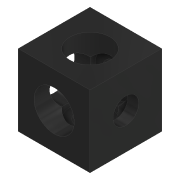
# Autodesk Inventor part: 2020CubeConnector
Saved by Autodesk Inventor 2020 (Build 240168000, 168)
## iProperties
Created: 2021-10-10
Part Number: 2020CubeConnector
Material: Aluminum 6061-AHC
Document SubType Name: Modeling
Designer: Henry Cawley
Density: 2.7 g/cm^3
Appearance: Aluminum - Dark(1)
Author: Henry Cawley
Autodesk Inventor part; units mm, degrees
ref_plane "YZ Plane" through (0, 0, 0) normal (1, 0, 0) x (0, 1, 0)
ref_plane "XZ Plane" through (0, 0, 0) normal (0, 1, 0) x (-1, 0, 0)
ref_plane "XY Plane" through (0, 0, 0) normal (0, 0, 1) x (1, 0, 0)
sketch "Sketch1" plane through (0, 0, 0) normal (1, 0, 0) x (0, 1, 0)
  line L0 (0, 0) -> (20, 0)
  line L1 (20, 0) -> (20, -20)
  line L2 (20, -20) -> (0, -20)
  line L3 (0, -20) -> (0, 0)
  dimension "d0" = 20
  dimension "d1" = 20
  constraints: 8 end point, 2 parallel, 1 horizontal, 1 perpendicular
  measures "d0" distance of L1.end L2.end
  measures "d1" distance of L0.end L1.end
extrude "Extrusion1" add sketch "Sketch1" along normal blind 20
sketch "Sketch2" plane through (0, 0, 0) normal (0, 0, 1) x (1, 0, 0)
  circle A0 centre (10, 10) radius 3.6
  line L0 (0, 20) -> (0, 0) projected
  line L1 (0, 20) -> (20, 20) projected
  dimension "d4" = 10
  dimension "d5" = 10
  dimension "d6" = 7.2
  constraints: 1 centre point
  measures "d4" distance from line of L0 A0.centre
  measures "d5" distance from line of A0.centre L1
  measures "d6" diameter of A0
extrude "Extrusion2" cut sketch "Sketch2" against normal blind 20
sketch "Sketch3" plane through (20, 0, 0) normal (1, 0, 0) x (0, 0, -1)
  circle A0 centre (10, 10) radius 3.6
  line L0 (20, 20) -> (0, 20) projected
  line L1 (0, 20) -> (0, 0) projected
  dimension "d9" = 10
  dimension "d10" = 10
  dimension "d11" = 7.2
  constraints: 1 centre point
  measures "d9" distance from line of L0 A0.centre
  measures "d10" distance from line of L1 A0.centre
  measures "d11" diameter of A0
extrude "Extrusion3" cut sketch "Sketch3" against normal blind 20
sketch "Sketch4" plane through (0, 20, 0) normal (0, 1, 0) x (1, 0, 0)
  line L0 (13.6, 6.4) -> (10, 10) projected
  circle A0 centre (10, 10) radius 3.6
  line L1 (20, 20) -> (20, 0) projected
  line L2 (0, 0) -> (20, 0) projected
  dimension "d14" = 7.2
  dimension "d15" = 10
  dimension "d16" = 10
  constraints: 1 centre point
  measures "d14" diameter of A0
  measures "d15" distance from line of L1 L0.end
  measures "d16" distance from line of L2 L0.end
extrude "Extrusion4" cut sketch "Sketch4" against normal blind 20
sketch "Sketch5" plane through (0, 0, 0) normal (-1, 0, 0) x (0, 0, 1)
  circle A0 centre (-10, 10) radius 3.6 projected
  circle A1 centre (-10, 10) radius 5.7
  point P0 (0, 0)
  dimension "d19" = 11.4
  constraints: 1 centre point, 1 coincident
  measures "d19" diameter of A1
extrude "Extrusion5" cut sketch "Sketch5" against normal blind 17 contours A0 | A1
sketch "Sketch6" plane through (0, 0, 0) normal (0, 0, 1) x (1, 0, 0)
  circle A0 centre (10, 10) radius 3.6 projected
  circle A1 centre (10, 10) radius 5.6
  point P0 (0, 0)
  dimension "d22" = 11.2
  constraints: 1 centre point, 1 coincident
  measures "d22" diameter of A1
extrude "Extrusion6" cut sketch "Sketch6" against normal blind 17 contours A0 | A1
sketch "Sketch7" plane through (0, 20, 0) normal (0, 1, 0) x (1, 0, 0)
  circle A0 centre (10, 10) radius 3.6 projected
  circle A1 centre (10, 10) radius 5.6
  point P0 (0, 0)
  dimension "d25" = 11.2
  constraints: 1 centre point, 1 coincident
  measures "d25" diameter of A1
extrude "Extrusion7" cut sketch "Sketch7" against normal blind 17 contours A0 | A1
body "Solid1"
